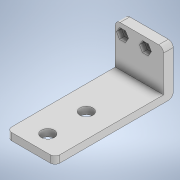
# Autodesk Inventor part: zupportenstop
Saved by Autodesk Inventor 2022 (Build 260153000, 153)
## iProperties
Created: 2022-03-19
Part Number: zupportenstop
Material: Genérico
Document SubType Name: Modeling
Designer: JK
Density: 1 g/cm^3
Appearance: Valor por defecto
Author: JK
Autodesk Inventor part; units mm, degrees
ref_plane "YZ Plane" through (0, 0, 0) normal (1, 0, 0) x (0, 1, 0)
ref_plane "XZ Plane" through (0, 0, 0) normal (0, 1, 0) x (-1, 0, 0)
ref_plane "XY Plane" through (0, 0, 0) normal (0, 0, 1) x (1, 0, 0)
sketch "Boceto1" plane through (0, 0, 0) normal (0, 1, 0) x (-1, 0, 0)
  line L0 (-10, 22.5) -> (10, 22.5)
  line L1 (10, 22.5) -> (10, -22.5)
  line L2 (10, -22.5) -> (-10, -22.5)
  line L3 (-10, -22.5) -> (-10, 22.5)
  line L4 (-10, 22.5) -> (10, -22.5) construction
  line L5 (10, 22.5) -> (-10, -22.5) construction
  circle A0 centre (0, 15.5) radius 2.7
  circle A1 centre (0, -0.5) radius 2.7
  point P0 (0, 0)
  point P1 (0, 0)
  dimension "d0" = 5.4
  dimension "d1" = 5.4
  dimension "d2" = 45
  dimension "d3" = 20
  dimension "d21" = 16
  dimension "d22" = 7
  constraints: 12 end point, 3 midpoint, 2 centre point, 2 parallel, 2 vertical alignment, 1 horizontal, 1 perpendicular
  measures "d0" diameter of A0
  measures "d1" diameter of A1
  measures "d2" distance of L0.end L1.end
  measures "d3" distance of L0.start L0.end
  measures "d21" distance of A1.centre A0.centre
  measures "d22" distance from line of L0 A0.centre
extrude "Extrusión1" add sketch "Boceto1" along normal blind 3
sketch "Boceto2" plane through (0, 0, 0) normal (0, -1, 0) x (1, 0, 0)
  line L0 (10, -22.5) -> (-10, -22.5) projected
  line L1 (10, -22.5) -> (-10, -22.5)
  line L2 (-10, -22.5) -> (-10, -26.5)
  line L3 (-10, -26.5) -> (10, -26.5)
  line L4 (10, -26.5) -> (10, -22.5)
  line L5 (-10, -22.5) -> (-10, 22.5) projected
  point P0 (0, 0)
  dimension "d8" = 4
  constraints: 8 end point, 2 parallel, 1 collinear, 1 horizontal, 1 perpendicular
  measures "d8" distance between parallel lines of L3 L0
extrude "Extrusión2" add sketch "Boceto2" against normal blind 20
sketch "Boceto3" plane through (10, 0, -26.5) normal (0, 0, -1) x (-1, 0, 0)
  circle A0 centre (7.5, 16) radius 1.2
  circle A1 centre (17, 16) radius 1.2
  line L0 (20, 0) -> (20, 20) projected
  line L1 (0, 20) -> (20, 20) projected
  point P0 (10, 0)
  dimension "d11" = 9.5
  dimension "d12" = 2.4
  dimension "d13" = 3
  dimension "d16" = 4
  constraints: 2 centre point, 1 equal radius, 1 horizontal alignment
  measures "d11" distance of A0.centre A1.centre
  measures "d12" diameter of A0
  measures "d13" distance from line of L0 A1.centre
  measures "d16" distance from line of L1 A0.centre
extrude "Extrusión3" cut sketch "Boceto3" against normal blind 20
sketch "Boceto4" plane through (-10, 3, -22.5) normal (0, 0, 1) x (1, 0, 0)
  circle A0 centre (12.5, 13) radius 1.2 projected
  line L0 (14.9826, 13) -> (13.7413, 10.85)
  line L1 (13.7413, 10.85) -> (11.2587, 10.85)
  line L2 (11.2587, 10.85) -> (10.0174, 13)
  line L3 (10.0174, 13) -> (11.2587, 15.15)
  line L4 (11.2587, 15.15) -> (13.7413, 15.15)
  line L5 (13.7413, 15.15) -> (14.9826, 13)
  circle A1 centre (3, 13) radius 1.2 projected
  line L6 (5.4826, 13) -> (4.2413, 10.85)
  line L7 (4.2413, 10.85) -> (1.7587, 10.85)
  line L8 (1.7587, 10.85) -> (0.5174, 13)
  line L9 (0.5174, 13) -> (1.7587, 15.15)
  line L10 (1.7587, 15.15) -> (4.2413, 15.15)
  line L11 (4.2413, 15.15) -> (5.4826, 13)
  circle A2 centre (12.5, 13) radius 2.15
  circle A3 centre (3, 13) radius 2.15
  point P0 (10, -3)
  dimension "d17" = 4.3
  constraints: 24 end point, 4 coincident, 2 centre point, 2 horizontal, 2 tangent, 1 equal radius, 26 other
  measures "d17" diameter of A2
extrude "Extrusión4" cut sketch "Boceto4" against normal blind 2 contours A0 | L0 A2 L5 | L0 L1 A2 | A2 | A2 L4 L5 | L1 L2 A2 | A2 L3 L4 | L2 L3 A2 | A1 | L6 A3 L11 | L6 L7 A3 | A3 | A3 L10 L11 | L7 L8 A3 | A3 L9 L10 | L8 L9 A3
fillet "Empalme1" radius 2 2 edges at (-10, 1.5, 22.5) (10, 1.5, 22.5)
fillet "Empalme2" radius 2 2 edges at (-10, 20, -24.5) (10, 20, -24.5)
fillet "Empalme3" radius 2 1 edges at (0, 0, -26.5)
